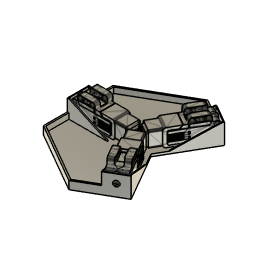
V1.2 RS WRO JSA v3 (Autodesk Fusion 360 design; units mm, degrees)
Autodesk Fusion 360 part; units mm, degrees
sketch "Dimensions" plane through (0, 0, 0) normal (0, 0, 1) x (1, 0, 0)
  line L0 (-100, 100) -> (100, 100)
  line L1 (100, 100) -> (100, -100)
  line L2 (100, -100) -> (-100, -100)
  line L3 (-100, -100) -> (-100, 100)
  constraint horizontal L0
  constraint vertical L1
  constraint horizontal L2
  constraint vertical L3
sketch "Hexagon" plane through (0, 0, 0) normal (0, 0, 1) x (1, 0, 0)
  line L0 (-75, -43.3013) -> (0, -86.6025)
  line L1 (0, -86.6025) -> (75, -43.3013)
  line L2 (75, -43.3013) -> (75, 43.3013)
  line L3 (75, 43.3013) -> (0, 86.6025)
  line L4 (0, 86.6025) -> (-75, 43.3013)
  line L5 (-75, 43.3013) -> (-75, -43.3013)
  dimension "d23" = 75
  measures "d23" distance of origin L5
other "Base Mesh Feature1"
extrude "Extrude1" add sketch "Hexagon" along normal blind 10 makes body 1
sketch "Sketch6" plane through (0, 0, 10) normal (0, 0, 1) x (-1, 0, 0)
  line L0 (-75, -43.3013) -> (0, -86.6025)
  line L1 (0, -86.6025) -> (75, -43.3013)
  line L2 (75, -43.3013) -> (75, 43.3013)
  line L3 (75, 43.3013) -> (0, 86.6025)
  line L4 (0, 86.6025) -> (-75, 43.3013)
  line L5 (-75, 43.3013) -> (-75, -43.3013)
  line L6 (0, 0) -> (-37.5, 64.9519)
  line L7 (0, 0) -> (75, 0)
  line L8 (0, 0) -> (-37.5, -64.9519)
  constraint coincident L6.start L7.start
  constraint midpoint L4 L6.end
  constraint midpoint L2 L7.end
  constraint midpoint L0 L8.end
other "Base Mesh Feature2"
sketch "--" plane through (0, 0, 10) normal (0, 0, 1) x (-1, 0, 0)
  line L0 (5, 8.6603) -> (-10, 0)
  line L1 (-10, 0) -> (5, -8.6603)
  line L2 (5, -8.6603) -> (5, 8.6603)
other "Modify2"
other "CopyPasteMeshes4"
other "Modify3"
other "CopyPasteMeshes5"
other "CopyPasteMeshes6"
other "Modify4"
extrude "Extrude2" add sketch "Hexagon" along normal blind 10 separate body makes body 2
sketch "---" plane through (0, 0, 10) normal (0, 0, 1) x (-1, 0, 0)
  line L0 (75, -43.3013) -> (75, 43.3013)
  line L1 (75, 43.3013) -> (0, 86.6025)
  line L2 (0, 86.6025) -> (-75, 43.3013)
  line L3 (-75, 43.3013) -> (-75, -43.3013)
  line L4 (-75, -43.3013) -> (0, -86.6025)
  line L5 (0, -86.6025) -> (75, -43.3013)
  line L6 (73, 42.1466) -> (0, 84.2931)
  line L7 (0, 84.2931) -> (-73, 42.1466)
  line L8 (-73, 42.1466) -> (-73, -42.1466)
  line L9 (-73, -42.1466) -> (0, -84.2931)
  line L10 (0, -84.2931) -> (73, -42.1466)
  line L11 (73, -42.1466) -> (73, 42.1466)
  dimension "d26" = 73
  measures "d26" distance of origin L11
extrude "Extrude3" cut sketch "---" against normal blind 7 contours L6 L7 L8 L9 L10 L11 bodies 2
sketch "SIde" plane through (-36.5, 63.2199, 0) normal (0.5, -0.866025, 0) x (0.866025, 0.5, 0)
  line L0 (42.1466, 10) -> (-42.1466, 10)
  line L1 (-42.1466, 10) -> (-42.1466, 3)
  line L2 (-42.1466, 3) -> (42.1466, 3)
  line L3 (42.1466, 3) -> (42.1466, 10)
  line L4 (0, 6.5) -> (0, 3)
  line L5 (0, 6.5) -> (12, 6.5)
  line L6 (0, 6.5) -> (-12, 6.5)
  line L7 (-12, 6.5) -> (-12, 13)
  line L8 (-12, 13) -> (12, 13)
  line L9 (12, 13) -> (12, 6.5)
  line L10 (-12, 6.5) -> (-12, 3)
  line L11 (12, 6.5) -> (12, 3)
  line L12 (12, 3) -> (-12, 3)
  dimension "d29" = 12
  dimension "d30" = 12
  constraint midpoint L2 L4.end
  constraint perpendicular L4 L5
  constraint horizontal L6
  constraint perpendicular L0 L7
  constraint perpendicular L7 L8
  constraint coincident L2 L10.end
  constraint perpendicular L2 L10
  constraint coincident L2 L11.end
  constraint perpendicular L2 L11
  measures "d29" distance of L4.start L5.end
  measures "d30" distance of L4.start L6.end
extrude "Extrude4" cut sketch "SIde" against normal blind 1 contours L0 L5 L6 L7 L9 | L2 L4 L5 L11 L12 | L2 L4 L6 L10 L12 bodies 2
sketch "----" plane through (0, 0, 10) normal (0, 0, 1) x (-1, 0, 0)
  line L0 (26.6077, -70.0859) -> (26.1077, -69.2199)
  line L1 (26.1077, -69.2199) -> (0, -84.2931)
  line L2 (0, -84.2931) -> (-73, -42.1466)
  line L3 (-73, -42.1466) -> (-73, 42.1466)
  line L4 (-73, 42.1466) -> (0, 84.2931)
  line L5 (0, 84.2931) -> (73, 42.1466)
  line L6 (73, 42.1466) -> (73, -42.1466)
  line L7 (73, -42.1466) -> (46.8923, -57.2199)
  line L8 (46.8923, -57.2199) -> (47.3923, -58.0859)
  line L9 (47.3923, -58.0859) -> (26.6077, -70.0859)
  line L10 (75, -43.3013) -> (75, 43.3013)
  line L11 (75, 43.3013) -> (0, 86.6025)
  line L12 (0, 86.6025) -> (-75, 43.3013)
  line L13 (-75, 43.3013) -> (-75, -43.3013)
  line L14 (-75, -43.3013) -> (0, -86.6025)
  line L15 (0, -86.6025) -> (75, -43.3013)
  line L16 (47.3923, -58.0859) -> (47.8923, -58.9519)
  line L17 (26.6077, -70.0859) -> (27.1077, -70.9519)
  line L18 (47.8923, -58.9519) -> (49.1913, -58.2019)
  line L19 (27.1077, -70.9519) -> (25.8087, -71.7019)
  line L20 (25.8087, -71.7019) -> (24.8087, -69.9699)
  line L21 (26.6077, -70.0859) -> (26.1077, -69.2199)
  line L22 (24.8087, -69.9699) -> (26.1077, -69.2199)
  line L23 (47.3923, -58.0859) -> (46.8923, -57.2199)
  line L24 (49.1913, -58.2019) -> (48.1913, -56.4699)
  line L25 (48.1913, -56.4699) -> (46.8923, -57.2199)
  dimension "d39" = 1.5
  dimension "d40" = 1.5
  constraint coincident L8.end L9.start
  constraint coincident L15 L16.end
  constraint perpendicular L15 L16
  constraint coincident L0.start L9.end
  constraint coincident L15 L17.end
  constraint perpendicular L15 L17
  constraint coincident L15 L18.end
  constraint coincident L15 L19.end
  constraint coincident L1 L20.end
  constraint perpendicular L1 L20
  constraint coincident L0.end L1.start
  constraint coincident L7.end L8.start
  constraint coincident L7 L24.end
  constraint perpendicular L7 L24
  measures "d39" distance of L16.end L18.end
  measures "d40" distance of L17.end L19.end
extrude "Extrude5" add sketch "----" along normal blind 15 contours L9 L15 L16 L17 bodies 2
sketch "Side" plane through (-37, 64.0859, 0) normal (0.5, -0.866025, 0) x (0.866025, 0.5, 0)
  line L0 (-12, 10) -> (-12, 3)
  line L1 (-12, 3) -> (12, 3)
  line L2 (12, 3) -> (12, 6.5)
  line L3 (12, 6.5) -> (12, 10)
  line L4 (12, 10) -> (12, 25)
  line L5 (12, 25) -> (-12, 25)
  line L6 (-12, 25) -> (-12, 10)
  line L7 (0, 3) -> (0, 11)
  line L8 (0, 18) -> (0, 11)
  circle A0 centre (0, 14.5) radius 3.5
  dimension "d35" = 8
  dimension "d36" = 15
  constraint midpoint L1 L7.start
  constraint perpendicular L1 L7
  constraint midpoint L8 A0.centre
  constraint coincident L7.end A0
  measures "d35" distance of L7.start L7.end
  measures "d36" distance of L7.start L8.start
extrude "Extrude6" cut sketch "Side" against normal blind 8 contours L8 A0 | L8 A0 bodies 2
extrude "Extrude7" add sketch "----" along normal blind 15 contours L0 L1 L15 L17 L19 L20 L21 L22 | L7 L8 L15 L16 L18 L23 L24 L25 bodies 2
sketch "-----" plane through (0, 0, 3) normal (0, 0, 1) x (-1, 0, 0)
  line L0 (73, -42.1466) -> (73, 42.1466)
  line L1 (73, 42.1466) -> (0, 84.2931)
  line L2 (0, 84.2931) -> (-73, 42.1466)
  line L3 (-73, 42.1466) -> (-73, -42.1466)
  line L4 (-73, -42.1466) -> (0, -84.2931)
  line L5 (0, -84.2931) -> (26.1077, -69.2199)
  line L6 (26.1077, -69.2199) -> (46.8923, -57.2199)
  line L7 (48.1913, -56.4699) -> (24.8087, -69.9699)
  line L8 (46.8923, -57.2199) -> (73, -42.1466)
sketch "Triangle 1" plane through (11.6913, 6.75, 0) normal (0.866025, 0.5, 0) x (-0.5, 0.866025, 0)
  line L0 (73, 10) -> (75, 10)
  line L1 (75, 10) -> (75, 25)
  line L2 (75, 25) -> (73, 25)
  line L3 (73, 25) -> (73, 10)
  line L4 (73, 25) -> (18.4564, 0)
  line L5 (18.4564, 0) -> (75, 0)
  line L6 (75, 0) -> (75, 25)
  dimension "d43" = 60
  constraint coincident L2.end L3.start
  constraint horizontal L5
  constraint coincident L1.end L2.start
  measures "d43" distance of L2.end L4.end
extrude "Extrude8" add sketch "Triangle 1" against normal blind 1.5 contours L0 L3 L4 L5 L6 bodies 2
sketch "Triangle 2" plane through (-11.6913, -6.75, 0) normal (-0.866025, -0.5, 0) x (0.5, -0.866025, 0)
  line L0 (-75, 10) -> (-73, 10)
  line L1 (-73, 10) -> (-73, 25)
  line L2 (-73, 25) -> (-75, 25)
  line L3 (-75, 25) -> (-75, 10)
  line L4 (-73, 25) -> (-73, 3)
  line L5 (-73, 3) -> (-73, 25)
  line L6 (-73, 25) -> (-25, 3)
  line L7 (-73, 3) -> (-25, 3)
  constraint coincident L1.end L2.start
  constraint perpendicular L2 L4
  constraint perpendicular L4 L7
extrude "Extrude9" add sketch "Triangle 2" against normal blind 1.5 contours L1 L4 L5 L6 L7 bodies 2
move_body "Move1" bodies 2 to x (0.866025, -0.5, 0) y (0.5, 0.866025, 0) z (0, 0, 1) at (0, 0, 0)
sketch "------" plane through (0, 0, 3) normal (0, 0, 1) x (-1, 0, 0)
move_body "Move2" bodies 2 to x (0.866025, 0.5, 0) y (-0.5, 0.866025, 0) z (0, 0, 1) at (0, 0, 0)
move_body "Move3" bodies 2 to x (0.5, 0.866025, 0) y (-0.866025, 0.5, 0) z (0, 0, 1) at (0, 0, 0)
other "Scale1"
sketch "-------" plane through (0, 0, 10) normal (0, 0, 1) x (-1, 0, 0)
  line L0 (75, -13.5) -> (73, -13.5)
  line L1 (73, -13.5) -> (73, -42.1466)
  line L2 (73, -42.1466) -> (0, -84.2931)
  line L3 (0, -84.2931) -> (-73, -42.1466)
  line L4 (-73, -42.1466) -> (-73, 42.1466)
  line L5 (-73, 42.1466) -> (0, 84.2931)
  line L6 (0, 84.2931) -> (73, 42.1466)
  line L7 (73, 42.1466) -> (73, 13.5)
  line L8 (73, 13.5) -> (75, 13.5)
  line L9 (75, 13.5) -> (75, 43.3013)
  line L10 (75, 43.3013) -> (0, 86.6025)
  line L11 (0, 86.6025) -> (-75, 43.3013)
  line L12 (-75, 43.3013) -> (-75, -43.3013)
  line L13 (-75, -43.3013) -> (0, -86.6025)
  line L14 (0, -86.6025) -> (75, -43.3013)
  line L15 (75, -43.3013) -> (75, -13.5)
  line L16 (37.5, 64.9519) -> (0, 0)
  line L17 (0, 0) -> (37.5, -64.9519)
  line L18 (0, 0) -> (-75, 0)
  constraint midpoint L10 L16.start
  constraint coincident L16.end L17.start
  constraint midpoint L14 L17.end
  constraint midpoint L12 L18.end
extrude "Extrude10" cut sketch "-------" against normal blind 10 contours L2 L3 L4 L12 L13 L14 L17 L18 | L2 L3 L4 L17 L18 | L4 L5 L6 L16 L18 | L4 L5 L6 L10 L11 L12 L16 L18 bodies 2
copy_body "CopyPasteBodies1" bodies 2 makes body 3
move_body "Move4" bodies 3 to x (-0.5, -0.866025, 0) y (0.866025, -0.5, 0) z (0, 0, 1) at (0, 0, 0)
copy_body "CopyPasteBodies2" bodies 3 makes body 4
move_body "Move5" bodies 4 to x (-0.5, -0.866025, 0) y (0.866025, -0.5, 0) z (0, 0, 1) at (0, 0, 0)
sketch "--------" plane through (0, 0, 3) normal (0, 0, 1) x (-1, 0, 0)
  line L0 (0, 0) -> (-73, 0)
  line L1 (-73, 0) -> (-73, -42.1466)
  line L2 (-73, -42.1466) -> (-48.1913, -56.4699)
  line L3 (-48.1913, -56.4699) -> (-24.1922, -14.9021)
  line L4 (-24.1922, -14.9021) -> (-22.8931, -15.6521)
  line L5 (-22.8931, -15.6521) -> (-46.8923, -57.2199)
  line L6 (-46.8923, -57.2199) -> (-26.1077, -69.2199)
  line L7 (-26.1077, -69.2199) -> (-2.1077, -27.6506)
  line L8 (-2.1077, -27.6506) -> (-0.8087, -28.4006)
  line L9 (-0.8087, -28.4006) -> (-24.8087, -69.9699)
  line L10 (-24.8087, -69.9699) -> (0, -84.2931)
  line L11 (0, -84.2931) -> (36.5, -63.2199)
  line L12 (36.5, -63.2199) -> (0, 0)
  circle A0 centre (0, 0) radius 5
  constraint coincident L0.start L12.end
extrude "Extrude11" add sketch "--------" against normal blind 1 contours L0 L12 A0 | L0 L12 A0 bodies 2 3 4
other "MeshRepair1"
other "MeshRepair2"
other "MeshRepair3"
other "MeshRepair4"
other "MeshRepair5"
ref_plane "WorkPlane1" through (36.6918, 36.552, 14) normal (0.866025, -0.5, 0) x (0.5, 0.866025, 0)
ref_plane "WorkPlane2" through (36.6913, -36.5513, 14) normal (0.866025, 0.5, 0) x (-0.5, 0.866025, 0)
split "Split1" by plane through (36.6918, 36.552, 14) normal (0.866025, -0.5, 0) bodies 2 makes body 5 at (32.7942, -18.9338, 0)
split "Split2" by plane through (36.6913, -36.5513, 14) normal (0.866025, 0.5, 0) bodies 5 makes body 6 at (55.1962, 0, 0)
combine "Combine1" operation add target body 2 tool bodies 5
hidden bodies 1 6
named bodies: "or hex", "final", "final (1)", "Extra block - no"
